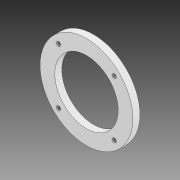
# Autodesk Inventor part: 2209B_Tube Flange Inner_V1
Saved by Autodesk Inventor 2020 (Build 240168000, 168)
## iProperties
Created: 2019-10-22
Part Number: 2209B_Tube Flange Inner_V1
Material: ABS Plastic
Document SubType Name: Modeling
Designer: RFLab
Density: 1.06 g/cm^3
Appearance: Smooth - White
Author: RFLab
Autodesk Inventor part; units mm, degrees
ref_plane "YZ Plane" through (0, 0, 0) normal (1, 0, 0) x (0, 1, 0)
ref_plane "XZ Plane" through (0, 0, 0) normal (0, 1, 0) x (-1, 0, 0)
ref_plane "XY Plane" through (0, 0, 0) normal (0, 0, 1) x (1, 0, 0)
sketch "Sketch8" plane through (0, 0, 0) normal (0, 0, 1) x (1, 0, 0)
  circle A0 centre (0, 0) radius 39.5
  circle A1 centre (0, 0) radius 27
  line L0 (-23.6881, -23.6881) -> (23.6881, -23.6881) construction
  line L1 (23.6881, -23.6881) -> (23.6881, 23.6881) construction
  line L2 (23.6881, 23.6881) -> (-23.6881, 23.6881) construction
  line L3 (-23.6881, 23.6881) -> (-23.6881, -23.6881) construction
  line L4 (-23.6881, -23.6881) -> (23.6881, 23.6881) construction
  line L5 (23.6881, -23.6881) -> (-23.6881, 23.6881) construction
  circle A2 centre (-23.6881, 23.6881) radius 1.75
  circle A3 centre (23.6881, 23.6881) radius 1.75
  circle A4 centre (-23.6881, -23.6881) radius 1.75
  circle A5 centre (23.6881, -23.6881) radius 1.75
  dimension "d23" = 79
  dimension "d24" = 54
  dimension "d25" = 67
  dimension "d26" = 3.5
  dimension "d27" = 3.5
  dimension "d28" = 3.5
  dimension "d29" = 3.5
  constraints: 12 end point, 6 centre point, 6 coincident, 2 midpoint, 2 parallel, 2 perpendicular, 1 horizontal
  measures "d23" diameter of A0
  measures "d24" diameter of A1
  measures "d25" distance of L0.start L1.end
  measures "d26" diameter of A2
  measures "d27" diameter of A5
  measures "d28" diameter of A3
  measures "d29" diameter of A4
extrude "Extrusion8" add sketch "Sketch8" along normal blind 6
equation "\"d27\" = d26"
equation "\"d28\" = d26"
equation "\"d29\" = d26"
body "Solid2"
